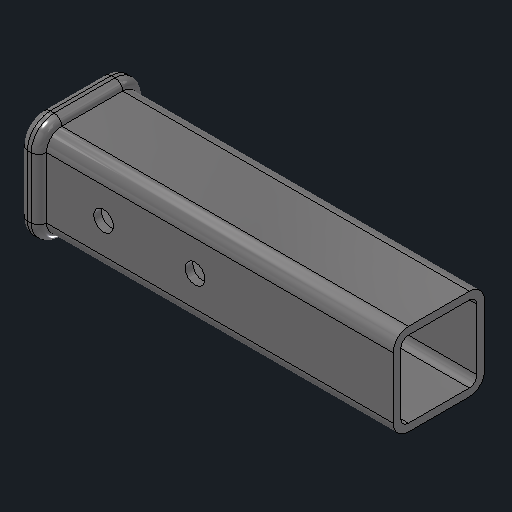
# Autodesk Inventor part: Front Hitch Model-1_Base Tube-2
Saved by Autodesk Inventor 2025.1 (Build 291241000, 241)
## iProperties
RuleStatus: InUse
Created: 2026-02-13
Part Number: Front Hitch Model-1_Base Tube-2
User Status: Released
Material: SS304
Description: Model-1 Base Tube-1
Document SubType Name: Modeling
Designer: Desktop -24
Density: 7.99949 g/cm^3
Appearance: Semi-Polished(1)
AfterDocNew0: Mat. Selection
encoded128: ÌStandard Î
encoded39: *STANDARD*
Family: SS304
Author: Desktop -24
Revision Number: 0
Autodesk Inventor part; units mm, degrees
ref_plane "YZ Plane" through (0, 0, 0) normal (1, 0, 0) x (0, 1, 0)
ref_plane "XZ Plane" through (0, 0, 0) normal (0, 1, 0) x (-1, 0, 0)
ref_plane "XY Plane" through (0, 0, 0) normal (0, 0, 1) x (1, 0, 0)
sketch "Sketch5" plane through (0, 0, 0) normal (1, 0, 0) x (0, 1, 0)
  line L0 (-25.4, 38.1) -> (25.4, 38.1)
  line L1 (38.1, 25.4) -> (38.1, -25.4)
  line L2 (25.4, -38.1) -> (-25.4, -38.1)
  line L3 (-38.1, -25.4) -> (-38.1, 25.4)
  line L4 (-38.1, 38.1) -> (38.1, -38.1) construction
  line L5 (38.1, 38.1) -> (-38.1, -38.1) construction
  arc A0 (38.1, 25.4) -> (25.4, 38.1) centre (25.4, 25.4) ccw
  arc A1 (25.4, -38.1) -> (38.1, -25.4) centre (25.4, -25.4) ccw
  arc A2 (-38.1, -25.4) -> (-25.4, -38.1) centre (-25.4, -25.4) ccw
  arc A3 (-25.4, 38.1) -> (-38.1, 25.4) centre (-25.4, 25.4) ccw
  line L6 (31.75, -25.4) -> (31.75, 25.4)
  arc A4 (31.75, 25.4) -> (25.4, 31.75) centre (25.4, 25.4) ccw
  line L7 (25.4, 31.75) -> (-25.4, 31.75)
  arc A5 (-25.4, 31.75) -> (-31.75, 25.4) centre (-25.4, 25.4) ccw
  line L8 (-31.75, 25.4) -> (-31.75, -25.4)
  arc A6 (-31.75, -25.4) -> (-25.4, -31.75) centre (-25.4, -25.4) ccw
  line L9 (-25.4, -31.75) -> (25.4, -31.75)
  arc A7 (25.4, -31.75) -> (31.75, -25.4) centre (25.4, -25.4) ccw
  point P0 (0, 0)
  dimension "d6" = 76.2
  dimension "d7" = 76.2
  dimension "d8" = 12.7
  dimension "d9" = 6.35
  constraints: 20 end point, 16 point on circle, 8 centre point, 8 point on line, 8 tangent, 4 parallel, 3 equal radius, 2 midpoint, 2 perpendicular, 1 horizontal, 7 other
  measures "d6" distance of L5.start L4.end
  measures "d7" distance of L4.end L5.end
  measures "d8" radius of A0
  measures "d9" distance between parallel lines of L1 L6
extrude "Extrusion4" add sketch "Sketch5" along normal mid plane 304.8
sketch "Sketch7" plane through (-152.4, 0, 0) normal (-1, 0, 0) x (0, 0, 1)
  arc A0 (-38.1, -25.4) -> (-25.4, -38.1) centre (-25.4, -25.4) ccw projected
  line L0 (-25.4, -38.1) -> (25.4, -38.1) projected
  arc A1 (25.4, -38.1) -> (38.1, -25.4) centre (25.4, -25.4) ccw projected
  line L1 (38.1, -25.4) -> (38.1, 25.4) projected
  arc A2 (38.1, 25.4) -> (25.4, 38.1) centre (25.4, 25.4) ccw projected
  line L2 (25.4, 38.1) -> (-25.4, 38.1) projected
  arc A3 (-25.4, 38.1) -> (-38.1, 25.4) centre (-25.4, 25.4) ccw projected
  line L3 (-38.1, 25.4) -> (-38.1, -25.4) projected
  arc A4 (-44.45, -25.4) -> (-25.4, -44.45) centre (-25.4, -25.4) ccw
  line L4 (-25.4, -44.45) -> (25.4, -44.45)
  arc A5 (25.4, -44.45) -> (44.45, -25.4) centre (25.4, -25.4) ccw
  line L5 (44.45, -25.4) -> (44.45, 25.4)
  arc A6 (44.45, 25.4) -> (25.4, 44.45) centre (25.4, 25.4) ccw
  line L6 (25.4, 44.45) -> (-25.4, 44.45)
  arc A7 (-25.4, 44.45) -> (-44.45, 25.4) centre (-25.4, 25.4) ccw
  line L7 (-44.45, 25.4) -> (-44.45, -25.4)
  point P0 (0, 0)
  constraints: 8 end point, 8 point on circle, 4 centre point, 7 other
extrude "Extrusion5" add sketch "Sketch7" against normal blind 15.875
fillet "Fillet1" radius 6.35 16 edges at (-152.4, 38.8704, -38.8704) (-152.4, 0, -44.45) (-152.4, -38.8704, -38.8704) (-152.4, -44.45, 0) (-152.4, -38.8704, 38.8704) (-152.4, 0, 44.45) (-152.4, 38.8704, 38.8704) (-152.4, 44.45, 0) (-136.525, 38.8704, 38.8704) (-136.525, 0, 44.45) (-136.525, -38.8704, 38.8704) (-136.525, -44.45, 0) (-136.525, -38.8704, -38.8704) (-136.525, 0, -44.45) (-136.525, 38.8704, -38.8704) (-136.525, 44.45, 0)
sketch "Sketch8" plane through (0, 0, 0) normal (0, 0, 1) x (1, 0, 0)
  circle A0 centre (-88.9, 0) radius 8.255
  line L0 (-152.4, 25.4) -> (-152.4, -25.4) projected
  point P0 (0, 0)
  dimension "d15" = 63.5
  dimension "d16" = 16.51
  constraints: 1 centre point
  measures "d15" distance from line of L0 A0.centre
  measures "d16" diameter of A0
extrude "Extrusion6" cut sketch "Sketch8" along normal through all both and the other way through all
pattern_linear "Rectangular Pattern1" count 2 spacing 76.2 along (1, 0, 0) of "Extrusion6"
body "Solid4"
